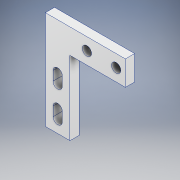
# Autodesk Inventor part: Gripper_Endstop_Holder
Saved by Autodesk Inventor 2021.3 (Build 253353000, 353)
## iProperties
Created: 2021-04-23
Part Number: Gripper_Endstop_Holder
Material: Aluminum 6061
Document SubType Name: Modeling
Designer: domin
Density: 2.7 g/cm^3
Appearance: Aluminum - Flat
Author: domin
Autodesk Inventor part; units mm, degrees
ref_plane "YZ Plane" through (0, 0, 0) normal (1, 0, 0) x (0, 1, 0)
ref_plane "XZ Plane" through (0, 0, 0) normal (0, 1, 0) x (-1, 0, 0)
ref_plane "XY Plane" through (0, 0, 0) normal (0, 0, 1) x (1, 0, 0)
sketch "Sketch1" plane through (0, 0, 0) normal (0, 0, 1) x (1, 0, 0)
  line L0 (-4, -24) -> (-4, 8)
  line L1 (-4, 8) -> (22, 8)
  line L2 (22, 8) -> (22, 0)
  line L3 (22, 0) -> (4, 0)
  line L4 (4, 0) -> (4, -24)
  line L5 (4, -24) -> (-4, -24)
  point P0 (0, 0)
  dimension "d0" = 0
  dimension "d1" = 8
  dimension "d2" = 8
  dimension "d3" = 4
  dimension "d5" = 26
  dimension "d6" = 32
  constraints: 12 end point, 5 perpendicular, 1 vertical
  measures "d0" distance from line of point (0, 0) L3
  measures "d1" distance between parallel lines of L3 L1
  measures "d2" distance of L4.end L0.start
  measures "d3" distance from line of point (0, 0) L0
  measures "d5" distance between parallel lines of L0 L2
  measures "d6" distance between parallel lines of L5 L1
extrude "Extrusion1" add sketch "Sketch1" along normal blind 3
sketch "Sketch2" plane through (0, 0, 3) normal (0, 0, 1) x (1, 0, 0)
  circle A0 centre (0, 4) radius 1.5
  circle A1 centre (19, 4) radius 1.5
  circle A2 centre (0, -6) radius 1.5
  circle A3 centre (9.5, 4) radius 1.5
  line L0 (-4, 8) -> (-4, -24) projected
  point P0 (0, 0)
  dimension "d9" = 3
  dimension "d10" = 3
  dimension "d11" = 3
  dimension "d12" = 10
  dimension "d15" = 4
  dimension "d24" = 9.5
  dimension "d25" = 13.5
  constraints: 4 centre point, 2 horizontal alignment, 2 vertical alignment, 1 equal radius
  measures "d9" diameter of A0
  measures "d10" diameter of A1
  measures "d11" diameter of A2
  measures "d12" distance of A0.centre A2.centre
  measures "d15" distance of point (0, 0) A0.centre
  measures "d24" distance of A1.centre A3.centre
  measures "d25" distance from line of L0 A3.centre
hole "Hole1" at (9.5, 4, 3) at (19, 4, 3) direction (0, 0, -1) diameter 3 end through all
sketch "Sketch3" plane through (0, 0, 3) normal (0, 0, 1) x (1, 0, 0)
  line L0 (0, -7) -> (0, -10) construction
  line L1 (-1.5, -7) -> (-1.5, -10)
  line L2 (1.5, -10) -> (1.5, -7)
  arc A0 (1.5, -7) -> (-1.5, -7) centre (0, -7) ccw
  arc A1 (-1.5, -10) -> (1.5, -10) centre (0, -10) ccw
  line L3 (0, -17) -> (0, -20) construction
  line L4 (-1.5, -17) -> (-1.5, -20)
  line L5 (1.5, -20) -> (1.5, -17)
  arc A2 (1.5, -17) -> (-1.5, -17) centre (0, -17) ccw
  arc A3 (-1.5, -20) -> (1.5, -20) centre (0, -20) ccw
  point P0 (0, 0)
  point P1 (0, -8.5)
  point P2 (0, -18.5)
  dimension "d26" = 3
  dimension "d27" = 3
  dimension "d29" = 10
  dimension "d32" = 7
  constraints: 16 end point, 8 point on circle, 8 tangent, 4 centre point, 2 midpoint, 2 parallel, 2 vertical, 2 vertical alignment, 1 collinear, 1 equal radius
  measures "d26" diameter of A1
  measures "d27" distance of L0.start L0.end
  measures "d29" distance of L3.start L0.start
  measures "d32" distance of point (0, 0) L0.start
extrude "Extrusion2" cut sketch "Sketch3" against normal through all
equation "\"d3\" = 0.5 * d2"
equation "\"d16\" = d11"
body "Solid1"
